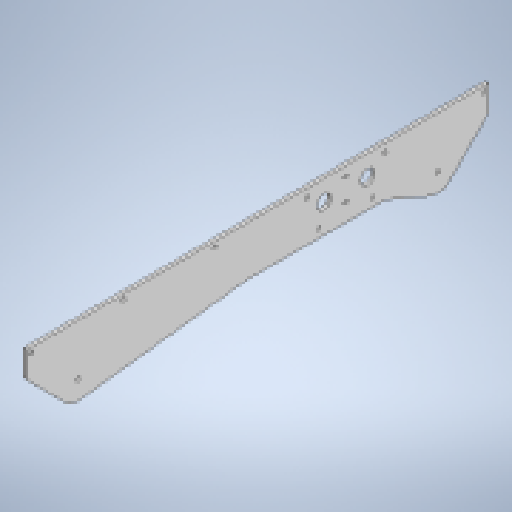
# Autodesk Inventor part: Outside Chassi Plate
Saved by Autodesk Inventor 2023 (Build 270158000, 158)
## iProperties
Created: 2022-09-05
Part Number: Outside Chassi Plate
Material: Generic
Document SubType Name: Modeling
Designer: deli
Density: 1 g/cm^3
Appearance: Default
Author: deli
Autodesk Inventor part; units mm, degrees
ref_plane "YZ Plane" through (0, 0, 0) normal (1, 0, 0) x (0, 1, 0)
ref_plane "XZ Plane" through (0, 0, 0) normal (0, 1, 0) x (-1, 0, 0)
ref_plane "XY Plane" through (0, 0, 0) normal (0, 0, 1) x (1, 0, 0)
sketch "Sketch1" plane through (0, 0, 0) normal (1, 0, 0) x (0, 1, 0)
  line L0 (-204.8959, 514.7923) -> (-204.8959, 64.7923)
  line L1 (-204.8959, 514.7923) -> (-229.8959, 514.7923)
  line L2 (-229.8959, 514.7923) -> (-267.5461, 477.5975)
  line L3 (-204.8959, 64.7923) -> (-229.8959, 64.7923)
  line L4 (-229.8959, 64.7923) -> (-267.5461, 101.9872)
  line L5 (-271.702, 121.2387) -> (-254.8959, 165.0535)
  line L6 (-254.8959, 165.0535) -> (-254.8959, 300.6153)
  line L7 (-254.8959, 300.6153) -> (-272.7873, 462.8188)
  circle A0 centre (-254.8959, 464.7923) radius 2
  arc A1 (-267.5461, 477.5975) -> (-272.7873, 462.8188) centre (-254.8959, 464.7923) ccw
  circle A2 centre (-254.8959, 464.7923) radius 48 construction
  arc A3 (-243.0401, 466.1792) -> (-266.7605, 463.4836) centre (-254.8959, 464.7923) ccw construction
  circle A4 centre (-254.8959, 114.7923) radius 48 construction
  arc A5 (-266.0407, 119.0672) -> (-243.8455, 110.2788) centre (-254.8959, 114.7923) ccw construction
  arc A6 (-271.702, 121.2387) -> (-267.5461, 101.9872) centre (-254.8959, 114.7923) ccw
  circle A7 centre (-254.8959, 114.7923) radius 2
  circle A8 centre (-227.6459, 225.0031) radius 7
  circle A9 centre (-227.6459, 183.6133) radius 7
  circle A10 centre (-227.6459, 225.0031) radius 18.75 construction
  circle A11 centre (-227.6459, 183.6133) radius 18.75 construction
  arc A12 (-240.3015, 223.6071) -> (-214.9997, 226.4825) centre (-227.6459, 225.0031) ccw construction
  arc A13 (-215.8588, 178.7989) -> (-239.5337, 188.1731) centre (-227.6459, 183.6133) ccw construction
  line L8 (-243.0401, 466.1792) -> (-214.9997, 226.4825) construction
  line L9 (-240.3015, 223.6071) -> (-266.7605, 463.4836) construction
  line L10 (-215.8588, 178.7989) -> (-243.8455, 110.2788) construction
  line L11 (-266.0407, 119.0672) -> (-239.5337, 188.1731) construction
  circle A14 centre (-209.8959, 240.0197) radius 2
  circle A15 centre (-210.6964, 204.3082) radius 2
  circle A16 centre (-244.5953, 204.3082) radius 2
  circle A17 centre (-249.3959, 233.2189) radius 2
  circle A18 centre (-249.3959, 175.3974) radius 2
  circle A19 centre (-209.8959, 168.5966) radius 2
  circle A20 centre (-209.8959, 509.7923) radius 2
  circle A21 centre (-209.8959, 69.7923) radius 2
  circle A22 centre (-209.8959, 419.8681) radius 2
  circle A23 centre (-209.8959, 329.9439) radius 2
  point P0 (0, 0)
  dimension "d43" = 450
  dimension "d44" = 4
  dimension "d45" = 36
  dimension "d46" = 96
  dimension "d47" = 23.8732
  dimension "d48" = 96
  dimension "d49" = 4
  dimension "d50" = 36
  dimension "d51" = 23.8732
  dimension "d52" = 50
  dimension "d53" = 50
  dimension "d54" = 50
  dimension "d55" = 50
  dimension "d56" = 25
  dimension "d57" = 25
  dimension "d58" = 14
  dimension "d59" = 14
  dimension "d60" = 37.5
  dimension "d61" = 37.5
  dimension "d62" = 25.4648
  dimension "d63" = 25.4648
  dimension "d64" = 179.622
  dimension "d65" = 179.622
  dimension "d66" = 178.768
  dimension "d67" = 178.768
  dimension "d68" = 241.3313
  dimension "d69" = 22.75
  dimension "d70" = 74.0152
  dimension "d71" = 22.75
  dimension "d72" = 50
  dimension "d73" = 4
  dimension "d74" = 4
  dimension "d75" = 4
  dimension "d77" = 4
  dimension "d78" = 4
  dimension "d90" = 6
  dimension "d91" = 6
  dimension "d92" = 6
  dimension "d93" = 6
  dimension "d94" = 2.5
  dimension "d95" = 2.5
  dimension "d96" = 2.5
  dimension "d97" = 2.5
  dimension "d98" = 5
  dimension "d99" = 5
  dimension "d100" = 90.913
  dimension "d103" = 4
  dimension "d104" = 4
  dimension "d105" = 4
  dimension "d106" = 4
  dimension "d107" = 5
  dimension "d108" = 5
  dimension "d109" = 5
  dimension "d110" = 5
  dimension "d111" = 5
  dimension "d112" = 5
  dimension "d113" = 269.7726
  dimension "d114" = 89.9242
  dimension "d115" = 89.9242
  dimension "d118" = 5.5
  dimension "d119" = 5.5
  dimension "d120" = 4
  constraints: 24 centre point, 24 end point, 12 point on circle, 12 tangent, 10 coincident, 2 parallel, 2 perpendicular, 2 vertical
  measures "d43" distance of L0.start L0.end
  measures "d44" diameter of A0
  measures "d45" diameter of A1
  measures "d46" diameter of A2
  measures "d47" diameter of A3
  measures "d48" diameter of A4
  measures "d49" diameter of A7
  measures "d50" diameter of A6
  measures "d51" diameter of A5
  measures "d52" distance from line of L0 A1.centre
  measures "d53" distance from line of L0 A4.centre
  measures "d54" distance from line of A0.centre L1
  measures "d55" distance from line of L3 A7.centre
  measures "d56" distance of L0.start L1.end
  measures "d57" distance of L0.end L3.end
  measures "d58" diameter of A8
  measures "d59" diameter of A9
  measures "d60" diameter of A10
  measures "d61" diameter of A11
  measures "d62" diameter of A12
  measures "d63" diameter of A13
  measures "d68" distance of L8.start L8.end
  measures "d69" distance from line of L0 A8.centre
  measures "d70" distance of L10.start L10.end
  measures "d71" distance from line of L0 A9.centre
  measures "d72" distance between parallel lines of L0 L6
  measures "d73" diameter of A14
  measures "d74" diameter of A17
  measures "d75" diameter of A16
  measures "d77" diameter of A15
  measures "d78" diameter of A19
  measures "d98" distance from line of L0 A14.centre
  measures "d99" distance from line of L0 A19.centre
  measures "d103" diameter of A20
  measures "d104" diameter of A22
  measures "d105" diameter of A23
  measures "d106" diameter of A21
  measures "d107" distance from line of L0 A20.centre
  measures "d108" distance from line of L1 A20.centre
  measures "d109" distance from line of L0 A22.centre
  measures "d110" distance from line of L0 A23.centre
  measures "d111" distance from line of L0 A21.centre
  measures "d112" distance from line of L3 A21.centre
  measures "d113" distance of A14.centre A20.centre
  measures "d114" distance of A22.centre A20.centre
  measures "d115" distance of A23.centre A22.centre
  measures "d118" distance from line of L6 A18.centre
  measures "d119" distance from line of L6 A17.centre
  measures "d120" diameter of A18
extrude "Extrusion1" add sketch "Sketch1" along normal blind 3.175
body "Solid1"
